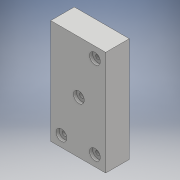
# Autodesk Inventor part: Housing Base
Saved by Autodesk Inventor 2017 (Build 210142000, 142)
## iProperties
Created: 2017-02-14
Part Number: Housing Base
Material: Generic
Document SubType Name: Modeling
Designer: William
Density: 1 g/cm^3
Appearance: Default
Author: William
Autodesk Inventor part; units mm, degrees
ref_plane "YZ Plane" through (0, 0, 0) normal (1, 0, 0) x (0, 1, 0)
ref_plane "XZ Plane" through (0, 0, 0) normal (0, 1, 0) x (-1, 0, 0)
ref_plane "XY Plane" through (0, 0, 0) normal (0, 0, 1) x (1, 0, 0)
sketch "Sketch1" plane through (0, 0, 0) normal (0, 1, 0) x (-1, 0, 0)
  circle A0 centre (0, 0) radius 1.6
  circle A1 centre (0, -62) radius 1.6
  circle A2 centre (25, -62) radius 1.6
  circle A3 centre (12, -31) radius 1.6
  circle A4 centre (12, -31) radius 2.5
  circle A5 centre (0, -62) radius 2.5
  circle A6 centre (25, -62) radius 2.5
  circle A7 centre (0, 0) radius 2.5
  line L0 (30, 5) -> (-5, 5)
  line L1 (-5, 5) -> (-5, -67)
  line L2 (-5, -67) -> (30, -67)
  line L3 (30, -67) -> (30, 5)
  line L4 (33, 8) -> (-8, 8)
  line L5 (-8, 8) -> (-8, -70)
  line L6 (-8, -70) -> (33, -70)
  line L7 (33, -70) -> (33, 8)
  dimension "d0" = 3.2
  dimension "d1" = 3.2
  dimension "d2" = 62
  dimension "d3" = 3.2
  dimension "d4" = 25
  dimension "d5" = 3.2
  dimension "d6" = 31
  dimension "d7" = 12
  dimension "d8" = 5
  dimension "d9" = 5
  dimension "d10" = 5
  dimension "d11" = 5
  dimension "d12" = 5
  dimension "d13" = 5
  dimension "d14" = 5
  dimension "d15" = 5
  dimension "d16" = 3
  dimension "d17" = 3
  dimension "d18" = 3
  dimension "d19" = 3
  dimension "d29" = 0
  constraints: 16 end point, 8 centre point, 5 coincident, 4 parallel, 2 horizontal, 2 perpendicular
  measures "d0" diameter of A0
  measures "d1" diameter of A1
  measures "d2" distance of point (0, 0) A1.centre
  measures "d3" diameter of A2
  measures "d4" distance of A1.centre A2.centre
  measures "d5" diameter of A3
  measures "d6" vertical distance of point (0, 0) A3.centre
  measures "d7" horizontal distance of point (0, 0) A3.centre
  measures "d8" diameter of A4
  measures "d9" diameter of A5
  measures "d10" diameter of A6
  measures "d11" diameter of A7
  measures "d12" distance from line of L2 A2.centre
  measures "d13" distance from line of A2.centre L3
  measures "d14" distance from line of L1 A0.centre
  measures "d15" distance from line of L0 point (0, 0)
  measures "d16" distance between parallel lines of L4 L0
  measures "d17" distance between parallel lines of L3 L7
  measures "d18" distance between parallel lines of L2 L6
  measures "d19" distance between parallel lines of L1 L5
  measures "d29" vertical distance of A1.centre A2.centre
extrude "Extrusion1" add sketch "Sketch1" along normal blind 12
sketch "Sketch2" plane through (0, 0, 0) normal (0, -1, 0) x (1, 0, 0)
  line L0 (-33, 8) -> (8, 8) projected
  line L1 (-33, -70) -> (-33, 8) projected
  line L2 (8, 8) -> (-33, 8)
  line L3 (-33, 8) -> (-33, -70)
  line L4 (-33, -70) -> (8, -70)
  line L5 (8, -70) -> (8, 8)
  point P0 (0, 0)
  constraints: 8 end point, 2 parallel, 1 horizontal, 1 perpendicular
extrude "Extrusion2" add sketch "Sketch2" along normal blind 4
sketch "Sketch3" plane through (0, 12, 0) normal (0, 1, 0) x (1, 0, 0)
  circle A0 centre (0, 0) radius 1.6 projected
  circle A1 centre (-12, 31) radius 1.6 projected
  circle A2 centre (-25, 62) radius 1.6 projected
  circle A3 centre (0, 62) radius 1.6 projected
extrude "Extrusion3" cut sketch "Sketch3" against normal up to next
sketch "Sketch4" plane through (0, -4, 0) normal (0, -1, 0) x (1, 0, 0)
  circle A0 centre (-25, -62) radius 1.6 projected
  circle A1 centre (-25, -62) radius 4
  circle A2 centre (0, -62) radius 1.6 projected
  circle A3 centre (0, -62) radius 4
  circle A4 centre (-12, -31) radius 1.6 projected
  circle A5 centre (-12, -31) radius 4
  circle A6 centre (0, 0) radius 1.6 projected
  circle A7 centre (0, 0) radius 4
  dimension "d26" = 8
  dimension "d27" = 8
  dimension "d28" = 8
  dimension "d30" = 8
  constraints: 4 centre point, 4 coincident
  measures "d26" diameter of A1
  measures "d27" diameter of A3
  measures "d28" diameter of A5
  measures "d30" diameter of A7
extrude "Extrusion4" cut sketch "Sketch4" against normal blind 2.2
sketch "Sketch6" plane through (0, 12, 0) normal (0, 1, 0) x (1, 0, 0)
  line L0 (-33, 70) -> (-33, -8) projected
  line L1 (8, 70) -> (-33, 70) projected
  line L2 (8, -8) -> (8, 70) projected
  line L3 (-33, -8) -> (8, -8) projected
  line L4 (-30, -5) -> (-30, 67) projected
  line L5 (5, -5) -> (-30, -5) projected
  line L6 (5, 67) -> (5, -5) projected
  line L7 (-30, 67) -> (5, 67) projected
  point P0 (0, 0)
extrude "Extrusion5" add sketch "Sketch6" along normal blind 1.6
sketch "Sketch7" plane through (0, 13.6, 0) normal (0, 1, 0) x (1, 0, 0)
  line L0 (-33, 70) -> (-33, -8) projected
  line L1 (-30, 67) -> (-30, -5) projected
  line L2 (-33, 20) -> (-30, 20)
  line L3 (-30, 20) -> (-30, 30)
  line L4 (-30, 30) -> (-33, 30)
  line L5 (-33, 30) -> (-33, 20)
  point P0 (0, 0)
  dimension "d35" = 20
  dimension "d36" = 10
  constraints: 8 end point, 2 parallel, 2 point on line, 1 horizontal, 1 perpendicular
  measures "d35" distance from line of L2 point (0, 0)
  measures "d36" distance between parallel lines of L2 L4
extrude "Extrusion6" cut sketch "Sketch7" against normal blind 2
body "Solid1"
